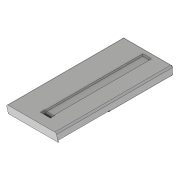
# Autodesk Inventor part: Temp
Saved by Autodesk Inventor 2021.2 (Build 252289000, 289)
## iProperties
Created: 2023-12-02
Part Number: Temp
Material: Типовые
Document SubType Name: Modeling
Designer: Egor
Density: 1 g/cm^3
Appearance: По умолчанию
Author: Egor
Autodesk Inventor part; units mm, degrees
ref_plane "YZ Plane" through (0, 0, 0) normal (1, 0, 0) x (0, 1, 0)
ref_plane "XZ Plane" through (0, 0, 0) normal (0, 1, 0) x (-1, 0, 0)
ref_plane "XY Plane" through (0, 0, 0) normal (0, 0, 1) x (1, 0, 0)
sketch "Эскиз1" plane through (0, 0, 0) normal (0, 1, 0) x (-1, 0, 0)
  line L0 (0, -50) -> (58, -50)
  line L1 (-2, -2) -> (-2, -48)
  line L2 (58, 0) -> (0, 0)
  line L3 (60, -48) -> (60, -2)
  line L4 (-2, 0) -> (60, 0)
  line L5 (60, 0) -> (60, -50)
  line L6 (60, -50) -> (-2, -50)
  line L7 (-2, -50) -> (-2, 0)
  circle A0 centre (2, -4) radius 1.6
  circle A1 centre (55, -4) radius 1.6
  circle A2 centre (55, -46) radius 1.6
  circle A3 centre (2, -46) radius 1.6
  circle A4 centre (2, -4) radius 1.6
  circle A5 centre (55, -4) radius 1.6
  circle A6 centre (55, -46) radius 1.6
  circle A7 centre (2, -46) radius 1.6
  circle A8 centre (2, -4) radius 2.4
  circle A9 centre (2, -4) radius 4
  circle A10 centre (55, -4) radius 4
  circle A11 centre (55, -4) radius 2.4
  circle A12 centre (55, -46) radius 4
  circle A13 centre (55, -46) radius 2.4
  circle A14 centre (2, -46) radius 4
  circle A15 centre (2, -46) radius 2.4
  dimension "d0" = 4.8
  dimension "d1" = 8
  dimension "d2" = 4.8
  dimension "d3" = 8
  dimension "d4" = 4.8
  dimension "d5" = 8
  dimension "d6" = 4.8
  dimension "d7" = 8
  constraints: 16 centre point, 16 end point, 9 coincident, 4 concentric, 2 parallel, 1 horizontal, 1 perpendicular, 1 point on line
  measures "d0" diameter of A8
  measures "d1" diameter of A9
  measures "d2" diameter of A11
  measures "d3" diameter of A10
  measures "d4" diameter of A13
  measures "d5" diameter of A12
  measures "d6" diameter of A15
  measures "d7" diameter of A14
extrude "Выдавливание1" add sketch "Эскиз1" along normal blind 2.5 contours L6 L7 L1 A14 L0 | A12 | A10 | A14 L1 A9 L2 L4 L5 L3 L6 L0 | A14 | L1 L7 L4 L2 A9 | A9 | A0 | A1 | A2 | A3 | A8 | A11 | A13 | A15
extrude "Выдавливание2" add sketch "Эскиз1" along normal blind 8.5 contours A12 | A10 | A14 | A9
sketch "Эскиз2" plane through (0, 0, 0) normal (0, -1, 0) x (1, 0, 0)
  line L0 (-60, 0) -> (2, 0) projected
  line L1 (2, 0) -> (2, -50) projected
  line L2 (2, -50) -> (-60, -50) projected
  line L3 (-60, -50) -> (-60, 0) projected
  line L4 (2, 0) -> (2, -50) projected
  line L5 (2.5, -50.5) -> (-60.5, -50.5)
  line L6 (-60.5, -50.5) -> (-60.5, 0.5)
  line L7 (-60.5, 0.5) -> (2.5, 0.5)
  line L8 (2.5, 0.5) -> (2.5, -50.5)
  line L9 (5, -50.5) -> (5, -53)
  line L10 (5, -53) -> (2.5, -53)
  line L11 (5, -53) -> (-63, -53)
  line L12 (-63, -53) -> (-63, 3)
  line L13 (-63, 3) -> (5, 3)
  line L14 (5, 3) -> (5, -53)
  point P0 (0, 0)
  dimension "d14" = 63
  dimension "d15" = 51
  dimension "d16" = 2.5
  dimension "d17" = 2.5
  dimension "d18" = 68
  dimension "d19" = 56
  constraints: 20 end point, 4 parallel, 2 horizontal, 2 perpendicular
  measures "d14" distance of L6.end L7.end
  measures "d15" distance of L5.end L6.end
  measures "d16" distance of L9.end L10.end
  measures "d17" distance of L9.start L9.end
  measures "d18" distance of L12.end L13.end
  measures "d19" distance of L11.end L12.end
extrude "Выдавливание3" add sketch "Эскиз2" against normal blind 2.5 contours L5 L6 L7 L8
extrude "Выдавливание4" add sketch "Эскиз2" against normal blind 35 contours L9 L10 L11 L12 L13 L14
sketch "Эскиз3" plane through (-63, 0, 3) normal (0, 0, 1) x (1, 0, 0)
  line L0 (0, 0) -> (0, 35) projected
  line L1 (0, 35) -> (68, 35)
  line L2 (68, 35) -> (68, 50)
  line L3 (68, 50) -> (0, 50)
  line L4 (0, 50) -> (0, 35)
  point P0 (63, 0)
  dimension "d24" = 15
  constraints: 8 end point, 2 parallel, 1 horizontal, 1 perpendicular
  measures "d24" distance of L2.end L1.end
extrude "Выдавливание5" add sketch "Эскиз3" against normal blind 150
sketch "Эскиз4" plane through (-63, 50, 3) normal (0, 1, 0) x (1, 0, 0)
  line L0 (0, 0) -> (0, 56) projected
  line L1 (68, 0) -> (68, 150) projected
  line L2 (0, 0) -> (68, 0)
  line L3 (68, 0) -> (68, 150)
  line L4 (68, 150) -> (0, 150)
  line L5 (0, 150) -> (0, 0)
  point P0 (63, 3)
  constraints: 8 end point, 2 parallel, 1 horizontal, 1 perpendicular
extrude "Выдавливание6" cut sketch "Эскиз4" against normal blind 2.5
sketch "Эскиз5" plane through (-63, 47.5, 3) normal (0, 1, 0) x (1, 0, 0)
  line L0 (0, 56) -> (0, 150) projected
  line L1 (0, 150) -> (10, 150)
  line L2 (10, 150) -> (10, 140)
  line L3 (10, 140) -> (0, 140)
  line L4 (0, 140) -> (0, 150)
  line L5 (68, 150) -> (0, 150) projected
  line L6 (68, 150) -> (58, 150)
  line L7 (58, 150) -> (58, 140)
  line L8 (58, 140) -> (68, 140)
  line L9 (68, 140) -> (68, 150)
  line L10 (0, 0) -> (0, 56) projected
  line L11 (0, 0) -> (10, 0)
  line L12 (10, 0) -> (10, 10)
  line L13 (10, 10) -> (0, 10)
  line L14 (0, 10) -> (0, 0)
  line L15 (10, 10) -> (58, 10)
  line L16 (58, 10) -> (58, 140)
  line L17 (58, 140) -> (10, 140)
  line L18 (10, 140) -> (10, 10)
  point P0 (63, 3)
  dimension "d29" = 10
  dimension "d30" = 10
  dimension "d31" = 10
  dimension "d32" = 10
  dimension "d33" = 10
  dimension "d34" = 10
  constraints: 32 end point, 8 parallel, 4 horizontal, 4 perpendicular
  measures "d29" distance of L2.end L3.end
  measures "d30" distance of L1.end L2.end
  measures "d31" distance of L8.end L7.end
  measures "d32" distance of L7.end L6.end
  measures "d33" distance of L13.end L12.end
  measures "d34" distance of L12.end L11.end
extrude "Выдавливание7" cut sketch "Эскиз5" against normal blind 10 contours L17 L16 L15 L18
sketch "Эскиз6" plane through (-63, 37.5, 3) normal (0, 1, 0) x (1, 0, 0)
  line L0 (58, 140) -> (10, 140) projected
  line L1 (10, 140) -> (10, 10) projected
  line L2 (10, 10) -> (58, 10) projected
  line L3 (58, 10) -> (58, 140) projected
  line L4 (0, 150) -> (68, 150) projected
  line L5 (68, 150) -> (68, 0) projected
  line L6 (68, 0) -> (0, 0) projected
  line L7 (0, 0) -> (0, 150) projected
  line L8 (68, 56) -> (0, 56) projected
  line L9 (0, 56) -> (10, 56)
  line L10 (10, 56) -> (10, 46)
  line L11 (10, 46) -> (0, 46)
  line L12 (0, 46) -> (0, 56)
  line L13 (10, 46) -> (58, 46)
  line L14 (58, 46) -> (58, 10)
  line L15 (58, 10) -> (10, 10)
  line L16 (10, 10) -> (10, 46)
  point P0 (63, 3)
  dimension "d37" = 10
  dimension "d38" = 10
  constraints: 16 end point, 4 parallel, 2 horizontal, 2 perpendicular
  measures "d37" distance of L10.end L11.end
  measures "d38" distance of L9.end L10.end
extrude "Выдавливание8" cut sketch "Эскиз6" against normal blind 10 contours L3 L2 L1 L13
sketch "Эскиз7" plane through (-63, 47.5, 3) normal (0, 1, 0) x (1, 0, 0)
  line L0 (0, 0) -> (0, 150) projected
  line L1 (0, 150) -> (2.5, 150)
  line L2 (2.5, 150) -> (2.5, 147.5)
  line L3 (2.5, 147.5) -> (0, 147.5)
  line L4 (0, 147.5) -> (0, 150)
  line L5 (68, 150) -> (68, 0) projected
  line L6 (68, 150) -> (65.5, 150)
  line L7 (65.5, 150) -> (65.5, 147.5)
  line L8 (65.5, 147.5) -> (68, 147.5)
  line L9 (68, 147.5) -> (68, 150)
  line L10 (2.5, 2.5) -> (2.5, 53.5) projected
  line L11 (65.5, 147.5) -> (2.5, 147.5)
  line L12 (2.5, 147.5) -> (2.5, 10)
  line L13 (2.5, 10) -> (65.5, 10)
  line L14 (65.5, 10) -> (65.5, 147.5)
  point P0 (63, 3)
  dimension "d41" = 2.5
  dimension "d42" = 2.5
  dimension "d43" = 2.5
  dimension "d44" = 2.5
  dimension "d45" = 137.5
  constraints: 24 end point, 6 parallel, 3 horizontal, 3 perpendicular, 1 point on line
  measures "d41" distance of L2.end L3.end
  measures "d42" distance of L1.end L2.end
  measures "d43" distance of L8.end L7.end
  measures "d44" distance of L7.end L6.end
  measures "d45" distance of L12.end L11.end
extrude "Выдавливание9" cut sketch "Эскиз7" against normal blind 10 contours L11 L14 L13 L10 L12
sketch "Эскиз8" plane through (-63, 37.5, 3) normal (0, 1, 0) x (1, 0, 0)
  line L0 (58, 10) -> (58, 46) projected
  line L1 (58, 46) -> (10, 46) projected
  line L2 (10, 46) -> (10, 10) projected
  line L3 (2.5, 10) -> (10, 10) projected
  line L4 (2.5, 147.5) -> (2.5, 10) projected
  line L5 (65.5, 147.5) -> (2.5, 147.5) projected
  line L6 (65.5, 10) -> (65.5, 147.5) projected
  line L7 (58, 10) -> (65.5, 10) projected
  line L8 (10, 10) -> (58, 10) projected
  line L9 (0, 150) -> (68, 150) projected
  line L10 (68, 150) -> (68, 0) projected
  line L11 (68, 0) -> (0, 0) projected
  line L12 (0, 0) -> (0, 150) projected
  circle A0 centre (8, 49) radius 2.4 projected
  line L13 (2.5, 53.5) -> (65.5, 53.5) projected
  line L14 (65.5, 147.5) -> (65.5, 10) projected
  circle A1 centre (61, 49) radius 4 projected
  circle A2 centre (8, 7) radius 4 projected
  circle A3 centre (8, 49) radius 4 projected
  line L15 (2.5, 2.5) -> (65.5, 2.5) projected
  line L16 (65.5, 2.5) -> (65.5, 53.5) projected
  line L17 (65.5, 53.5) -> (2.5, 53.5) projected
  line L18 (2.5, 53.5) -> (2.5, 2.5) projected
  circle A4 centre (61, 7) radius 4 projected
  circle A5 centre (8, 7) radius 4 projected
  line L19 (2.5, 2.5) -> (2.5, 53.5) projected
  line L20 (65.5, 2.5) -> (2.5, 2.5) projected
  line L21 (65.5, 53.5) -> (65.5, 2.5) projected
  circle A6 centre (61, 7) radius 2.4 projected
  line L22 (2.5, 53.5) -> (65.5, 53.5)
  line L23 (65.5, 53.5) -> (65.5, 2.5)
  line L24 (65.5, 2.5) -> (2.5, 2.5)
  line L25 (2.5, 2.5) -> (2.5, 53.5)
  point P0 (63, 3)
  point P1 (58.3542, 10)
  point P2 (63.6458, 10)
  point P3 (10.6458, 10)
  point P4 (10, 10.4641)
  point P5 (10, 45.5359)
  point P6 (10.6458, 46)
  constraints: 8 end point, 2 parallel, 1 horizontal, 1 perpendicular
extrude "Выдавливание10" cut sketch "Эскиз8" along normal mid plane 20 contours L0 L1 A3 L2 A2 L3 L4 L13 L6 L7 A4 | L7 A4 L16 L15 L18 L3 A2 L8 | A4 L7 | L7 A4 | A2 L3 L8 | L8 L2 A2 | A3 L2 L1 | L1 L2 A3 | L3 A2 L2 | A0 | A1 | A6
sketch "Эскиз9" plane through (-63, 0, 3) normal (0, 0, 1) x (1, 0, 0)
  line L0 (68, 0) -> (68, 47.5) projected
  line L1 (68, 35) -> (0, 35) projected
  line L2 (68, 47.5) -> (0, 47.5)
  line L3 (0, 47.5) -> (0, 35)
  line L4 (0, 35) -> (68, 35)
  line L5 (68, 35) -> (68, 47.5)
  point P0 (63, 0)
  constraints: 8 end point, 2 parallel, 1 horizontal, 1 perpendicular
extrude "Выдавливание11" add sketch "Эскиз9" along normal blind 10
sketch "Эскиз12" plane through (-63, 37.5, 3) normal (0, 1, 0) x (1, 0, 0)
  line L0 (65.5, 2.5) -> (65.5, 53.5) projected
  line L1 (65.5, 53.5) -> (55.5, 53.5)
  line L2 (55.5, 53.5) -> (55.5, 63.5)
  line L3 (55.5, 63.5) -> (65.5, 63.5)
  line L4 (65.5, 63.5) -> (65.5, 53.5)
  line L5 (2.5, 53.5) -> (2.5, 2.5) projected
  line L6 (2.5, 53.5) -> (12.5, 53.5)
  line L7 (12.5, 53.5) -> (12.5, 63.5)
  line L8 (12.5, 63.5) -> (2.5, 63.5)
  line L9 (2.5, 63.5) -> (2.5, 53.5)
  point P0 (63, 3)
  dimension "d52" = 10
  dimension "d53" = 10
  dimension "d54" = 10
  constraints: 16 end point, 4 parallel, 2 horizontal, 2 perpendicular
  measures "d52" distance of L2.end L3.end
  measures "d53" distance of L1.end L2.end
  measures "d54" distance of L8.end L7.end
extrude "Выдавливание12" add sketch "Эскиз12" along normal blind 10
sketch "Эскиз16" plane through (0, 0, 0) normal (0, -1, 0) x (1, 0, 0)
  line L0 (5, -53) -> (5, 3) projected
  line L1 (-63, -53) -> (5, -53) projected
  line L2 (5, 3) -> (-63, 3)
  line L3 (-63, 3) -> (-63, -53)
  line L4 (-63, -53) -> (5, -53)
  line L5 (5, -53) -> (5, 3)
  line L6 (-63, -147) -> (-63, 13) projected
  line L7 (5, -53) -> (-63, -53)
  line L8 (-63, -53) -> (-63, -60)
  line L9 (-63, -60) -> (5, -60)
  line L10 (5, -60) -> (5, -53)
  line L11 (-63, 3) -> (-63, -53) projected
  line L12 (5, -147) -> (5, 13) projected
  line L13 (-63, 3) -> (5, 3)
  line L14 (5, 3) -> (5, 10)
  line L15 (5, 10) -> (-63, 10)
  line L16 (-63, 10) -> (-63, 3)
  point P0 (0, 0)
  dimension "d59" = 7
  dimension "d60" = 7
  constraints: 24 end point, 6 parallel, 3 horizontal, 3 perpendicular, 2 point on line
  measures "d59" distance of L8.end L7.end
  measures "d60" distance of L14.end L13.end
extrude "Выдавливание13" cut sketch "Эскиз16" against normal blind 37.5
sketch "Эскиз17" plane through (-63, 47.5, 3) normal (0, 1, 0) x (1, 0, 0)
  line L0 (68, -10) -> (0, -10)
  line L1 (0, -10) -> (0, 150)
  line L2 (0, 150) -> (68, 150)
  line L3 (68, 150) -> (68, -10)
  line L4 (45.5, 63.5) -> (45.5, 127.5)
  line L5 (2.5, 147.5) -> (65.5, 147.5) projected
  line L6 (45.5, 127.5) -> (45.5, 132.5)
  line L7 (33.5, 132.5) -> (33.5, 7.5)
  line L8 (33.5, 7.5) -> (45.5, 7.5)
  line L9 (45.5, 7.5) -> (45.5, 63.5)
  line L10 (33.5, 132.5) -> (32, 132.5)
  line L11 (32, 132.5) -> (32, 134)
  line L12 (32, 134) -> (33.5, 134)
  line L13 (33.5, 134) -> (33.5, 132.5)
  line L14 (45.5, 7.5) -> (47, 7.5)
  line L15 (47, 7.5) -> (47, 6)
  line L16 (47, 6) -> (45.5, 6)
  line L17 (45.5, 6) -> (45.5, 7.5)
  line L18 (47, 6) -> (32, 6)
  line L19 (32, 6) -> (32, 134)
  line L20 (47, 134) -> (47, 6)
  line L21 (45.5, 134) -> (45.5, 132.5)
  line L22 (33.5, 132.5) -> (33.5, 134)
  line L23 (47, 134) -> (47, 144)
  line L24 (47, 144) -> (32, 144)
  line L25 (32, 144) -> (32, 134)
  line L26 (33.5, 134) -> (32, 134)
  line L27 (32, 134) -> (32, 144)
  line L28 (32, 144) -> (33.5, 144)
  line L29 (33.5, 144) -> (33.5, 134)
  line L30 (45.5, 134) -> (47, 134)
  line L31 (47, 134) -> (47, 144)
  line L32 (47, 144) -> (45.5, 144)
  line L33 (45.5, 144) -> (45.5, 134)
  line L34 (32, 144) -> (47, 144)
  line L35 (47, 144) -> (47, 142.5)
  line L36 (47, 142.5) -> (32, 142.5)
  line L37 (32, 142.5) -> (32, 144)
  line L38 (32, 6) -> (47, 6)
  line L39 (47, 6) -> (47, 7.5)
  line L40 (47, 7.5) -> (32, 7.5)
  line L41 (32, 7.5) -> (32, 6)
  point P0 (63, 3)
  point P1 (55.5, 63.5)
  point P2 (33.5, 142.5)
  point P3 (45.5, 142.5)
  dimension "d64" = 64
  dimension "d65" = 5
  dimension "d66" = 12
  dimension "d67" = 125
  dimension "d68" = 1.5
  dimension "d69" = 1.5
  dimension "d70" = 1.5
  dimension "d71" = 1.5
  dimension "d72" = 10
  dimension "d73" = 1.5
  constraints: 82 end point, 17 parallel, 11 perpendicular, 8 horizontal, 3 point on line
  measures "d64" distance of L4.start L4.end
  measures "d65" distance of L4.end L6.end
  measures "d66" distance of L6.end L7.start
  measures "d67" distance of L7.start L7.end
  measures "d68" distance of L11.end L12.end
  measures "d69" distance of L10.end L11.end
  measures "d70" distance of L15.end L16.end
  measures "d71" distance of L14.end L15.end
  measures "d72" distance of L23.end L23.start
  measures "d73" distance of L34.end L35.end
extrude "Выдавливание14" add sketch "Эскиз17" against normal up to surface (10 mm away) contours L4 L6 L21 L30 L20 L14 L9 | L40 L19 L10 L7 | L33 L36 L23 L30 | L10 L11 L12 L13 | L36 L29 L24 L33 | L33 L24 L23 L36 | L12 L25 L36 L29 | L36 L25 L24 L29
sketch "Эскиз18" plane through (-63, 37.5, 3) normal (0, 1, 0) x (1, 0, 0)
  line L0 (45.5, 142.5) -> (45.5, 7.5) projected
  line L1 (33.5, 142.5) -> (45.5, 142.5)
  line L2 (45.5, 142.5) -> (45.5, 7.5)
  line L3 (45.5, 7.5) -> (33.5, 7.5)
  line L4 (33.5, 7.5) -> (33.5, 142.5)
  point P0 (63, 3)
  constraints: 8 end point, 2 parallel, 1 horizontal, 1 perpendicular
extrude "Выдавливание15" add sketch "Эскиз18" along normal blind 7.5
sketch "Эскиз19" plane through (-63, 47.5, 3) normal (0, 1, 0) x (1, 0, 0)
  line L0 (68, 150) -> (0, 150) projected
  line L1 (68, 150) -> (68, -10) projected
  line L2 (0, 150) -> (68, 150)
  line L3 (68, 150) -> (68, -10)
  line L4 (68, -10) -> (0, -10)
  line L5 (0, -10) -> (0, 150)
  point P0 (63, 3)
  constraints: 8 end point, 2 parallel, 1 horizontal, 1 perpendicular
sketch "Эскиз20" plane through (-63, 37.5, 3) normal (0, 1, 0) x (1, 0, 0)
  line L0 (2.5, 147.5) -> (65.5, 147.5) projected
  line L1 (32, 63) -> (32, 7.5) projected
  line L2 (2.5, 147.5) -> (32, 147.5)
  line L3 (32, 147.5) -> (32, 63)
  line L4 (32, 63) -> (2.5, 63)
  line L5 (2.5, 63) -> (2.5, 147.5)
  line L6 (47, 7.5) -> (47, 144) projected
  line L7 (32, 147.5) -> (47, 147.5)
  line L8 (47, 147.5) -> (47, 144)
  line L9 (47, 144) -> (32, 144)
  line L10 (32, 144) -> (32, 147.5)
  line L11 (47, 147.5) -> (65.5, 147.5)
  line L12 (65.5, 147.5) -> (65.5, 63)
  line L13 (65.5, 63) -> (47, 63)
  line L14 (47, 63) -> (47, 147.5)
  point P0 (63, 3)
  constraints: 24 end point, 6 parallel, 3 horizontal, 3 perpendicular, 1 point on line
extrude "Выдавливание16" add sketch "Эскиз20" along normal blind 10
sketch "Эскиз21" plane through (-63, 47.5, 3) normal (0, 1, 0) x (1, 0, 0)
  line L0 (12.5, 63) -> (32, 63) projected
  line L1 (65.5, 2.5) -> (2.5, 2.5) projected
  line L2 (32, 63) -> (2.5, 63)
  line L3 (2.5, 63) -> (2.5, 2.5)
  line L4 (2.5, 2.5) -> (32, 2.5)
  line L5 (32, 2.5) -> (32, 63)
  line L6 (47, 63) -> (55.5, 63) projected
  line L7 (65.5, 53.5) -> (65.5, 2.5) projected
  line L8 (47, 63) -> (65.5, 63)
  line L9 (65.5, 63) -> (65.5, 2.5)
  line L10 (65.5, 2.5) -> (47, 2.5)
  line L11 (47, 2.5) -> (47, 63)
  line L12 (32, 2.5) -> (47, 2.5)
  line L13 (47, 2.5) -> (47, 5.5)
  line L14 (47, 5.5) -> (32, 5.5)
  line L15 (32, 5.5) -> (32, 2.5)
  point P0 (63, 3)
  dimension "d80" = 3
  constraints: 24 end point, 6 parallel, 3 horizontal, 3 perpendicular, 1 point on line
  measures "d80" distance of L13.end L12.end
extrude "Выдавливание17" add sketch "Эскиз21" against normal blind 10
sketch "Эскиз22" plane through (0, 37.5, 0) normal (0, -1, 0) x (1, 0, 0)
  line L0 (-16, -4.5) -> (-16, -2.5) projected
  line L1 (-16, -2.5) -> (-31, -2.5)
  line L2 (-31, -2.5) -> (-31, 0)
  line L3 (-31, 0) -> (-16, 0)
  line L4 (-16, 0) -> (-16, -2.5)
  point P0 (0, 0)
  constraints: 8 end point, 2 parallel, 1 horizontal, 1 perpendicular
extrude "Выдавливание18" cut sketch "Эскиз22" against normal blind 10
sketch "Эскиз23" plane through (-63, 47.5, 3) normal (0, 1, 0) x (1, 0, 0)
  line L0 (33.5, 7.5) -> (45.5, 7.5) projected
  line L1 (45.5, 142.5) -> (45.5, 7.5) projected
  line L2 (33.5, 7.5) -> (45.5, 7.5)
  line L3 (45.5, 7.5) -> (45.5, 9.5)
  line L4 (45.5, 9.5) -> (33.5, 9.5)
  line L5 (33.5, 9.5) -> (33.5, 7.5)
  point P0 (63, 3)
  dimension "d85" = 2
  constraints: 8 end point, 2 parallel, 1 horizontal, 1 perpendicular, 1 point on line
  measures "d85" distance of L3.end L2.end
extrude "Выдавливание19" cut sketch "Эскиз23" against normal blind 10
sketch "Эскиз24" plane through (-63, 47.5, 3) normal (0, 1, 0) x (1, 0, 0)
  line L0 (32, 7.5) -> (33.5, 7.5) projected
  line L1 (47, 3) -> (32, 3) projected
  line L2 (33.5, 7.5) -> (32, 7.5)
  line L3 (32, 7.5) -> (32, 3)
  line L4 (32, 3) -> (33.5, 3)
  line L5 (33.5, 3) -> (33.5, 7.5)
  line L6 (45.5, 7.5) -> (47, 7.5) projected
  line L7 (45.5, 7.5) -> (47, 7.5)
  line L8 (47, 7.5) -> (47, 3)
  line L9 (47, 3) -> (45.5, 3)
  line L10 (45.5, 3) -> (45.5, 7.5)
  point P0 (63, 3)
  constraints: 16 end point, 4 parallel, 2 horizontal, 2 perpendicular, 1 point on line
extrude "Выдавливание20" add sketch "Эскиз24" against normal blind 10
sketch "Эскиз25" plane through (-63, 47.5, 3) normal (0, 1, 0) x (1, 0, 0)
  line L0 (33.5, 3) -> (33.5, 142.5) projected
  line L1 (45.5, 142.5) -> (45.5, 3) projected
  line L2 (33.5, 3) -> (45.5, 3)
  line L3 (45.5, 3) -> (45.5, 10.5)
  line L4 (45.5, 10.5) -> (33.5, 10.5)
  line L5 (33.5, 10.5) -> (33.5, 3)
  point P0 (63, 3)
  dimension "d90" = 7.5
  constraints: 8 end point, 2 parallel, 1 horizontal, 1 perpendicular, 1 point on line
  measures "d90" distance of L3.end L2.end
extrude "Выдавливание21" add sketch "Эскиз25" against normal blind 1
sketch "Эскиз26" plane through (0, 37.5, 0) normal (0, -1, 0) x (1, 0, 0)
  point P0 (0, 0)
sketch "Эскиз27" plane through (0, 37.5, 0) normal (0, -1, 0) x (1, 0, 0)
  line L0 (-29.5, 0) -> (-29.5, -6.5) projected
  line L1 (-29.5, -6.5) -> (-17.5, -6.5) projected
  line L2 (-17.5, -6.5) -> (-17.5, 0) projected
  line L3 (-17.5, 0) -> (-29.5, 0) projected
  line L4 (-63, -60) -> (5, -60) projected
  line L5 (5, 10) -> (5, -60) projected
  line L6 (5, 13) -> (5, 10) projected
  line L7 (-63, 13) -> (5, 13) projected
  line L8 (-63, 10) -> (-63, 13) projected
  line L9 (5, 10) -> (-63, 10) projected
  line L10 (-63, -60) -> (-63, 10) projected
  line L11 (-63, -147) -> (-63, -60) projected
  line L12 (5, -147) -> (-63, -147) projected
  line L13 (5, -60) -> (5, -147) projected
  line L14 (5, 10) -> (-2, 10)
  line L15 (-2, 10) -> (-2, 3)
  line L16 (-2, 3) -> (5, 3)
  line L17 (5, 3) -> (5, 10)
  line L18 (-63, 10) -> (-56, 10)
  line L19 (-56, 10) -> (-56, 3)
  line L20 (-56, 3) -> (-63, 3)
  line L21 (-63, 3) -> (-63, 10)
  line L22 (-63, -60) -> (-56, -60)
  line L23 (-56, -60) -> (-56, -53)
  line L24 (-56, -53) -> (-63, -53)
  line L25 (-63, -53) -> (-63, -60)
  line L26 (5, -60) -> (-63, -60) projected
  line L27 (5, -60) -> (-2, -60)
  line L28 (-2, -60) -> (-2, -53)
  line L29 (-2, -53) -> (5, -53)
  line L30 (5, -53) -> (5, -60)
  circle A0 centre (-2, -56.5) radius 2.4
  circle A1 centre (-56, -56.5) radius 2.4
  circle A2 centre (-56, 6.5) radius 2.4
  circle A3 centre (-2, 6.5) radius 2.4
  point P0 (0, 0)
  dimension "d93" = 7
  dimension "d94" = 7
  dimension "d95" = 7
  dimension "d96" = 7
  dimension "d97" = 4.8
  constraints: 32 end point, 8 parallel, 4 centre point, 4 horizontal, 4 midpoint, 4 perpendicular, 4 point on line
  measures "d93" distance of L16.end L15.end
  measures "d94" distance of L15.end L14.end
  measures "d95" distance of L19.end L20.end
  measures "d96" distance of L23.end L22.end
  measures "d97" diameter of A0
extrude "Выдавливание22" cut sketch "Эскиз27" against normal blind 6 contours A1 L23 | L23 A1 | A0 L28 | L28 A0 | A2 L19 | L19 A2 | A3 L15 | L15 A3
sketch "Эскиз28" plane through (5, 35, -147) normal (1, 0, 0) x (0, 0, -1)
  line L0 (-160, 0) -> (-160, 12.5)
  line L1 (-150, -35) -> (-160, 0)
  line L2 (-150, -35) -> (-160, 12.5)
  line L3 (-160, 0) -> (-150, -35)
  line L4 (-160, 12.5) -> (-160, 0) projected
  line L5 (0, 12.5) -> (-160, 12.5) projected
  point P0 (-147, -35)
  constraints: 8 end point
extrude "Выдавливание23" cut sketch "Эскиз28" against normal through all
fillet "Сопряжение1" radius 2 8 edges at (5, 47.5, -67) (-29, 47.5, -147) (-63, 47.5, -67) (5, 41.25, -147) (-63, 41.25, -147) (-29, 35, -147) (5, 35, -103.5) (-63, 35, -103.5)
fillet "Сопряжение2" radius 2 1 edges at (-23.5, 45, -6.5)
fillet "Сопряжение3" radius 2 4 edges at (-23.5, 37.5, -6.5) (-17.5, 37.5, -3.25) (-29.5, 37.5, -3.25) (-23.5, 37.5, 0)
sketch "Эскиз29" plane through (0, 37.5, 0) normal (0, -1, 0) x (1, 0, 0)
  line L0 (-31.5, -8.5) -> (-29.5, -6.5) projected
  line L1 (-31.5, -8.5) -> (-31.5, -28.5)
  line L2 (-31.5, -28.5) -> (-15.5, -28.5)
  line L3 (-15.5, -28.5) -> (-15.5, -22.5)
  line L4 (-15.5, -22.5) -> (-31.5, -22.5)
  line L5 (-31.5, -28.5) -> (-28.5, -28.5)
  line L6 (-28.5, -28.5) -> (-28.5, -22.5)
  line L7 (-28.5, -22.5) -> (-31.5, -22.5)
  line L8 (-31.5, -22.5) -> (-31.5, -28.5)
  point P0 (0, 0)
  dimension "d105" = 20
  dimension "d106" = 3
  constraints: 16 end point, 3 perpendicular, 2 horizontal, 2 parallel, 2 point on line, 1 vertical
  measures "d105" distance of L0.start L1.end
  measures "d106" distance of L7.end L6.end
extrude "Выдавливание24" add sketch "Эскиз29" along normal blind 5 contours L4 L6 L2 L1
sketch "Эскиз30" plane through (0, 32.5, 0) normal (0, -1, 0) x (1, 0, 0)
  line L0 (-31.5, -28.5) -> (-31.5, -22.5) projected
  line L1 (-31.5, -28.5) -> (-16.5, -28.5)
  line L2 (-16.5, -28.5) -> (-16.5, -22.5)
  line L3 (-16.5, -22.5) -> (-31.5, -22.5)
  line L4 (-31.5, -22.5) -> (-31.5, -28.5)
  point P0 (0, 0)
  dimension "d109" = 15
  constraints: 8 end point, 2 parallel, 1 horizontal, 1 perpendicular
  measures "d109" distance of L3.end L2.end
extrude "Выдавливание25" add sketch "Эскиз30" against normal blind 2
fillet "Сопряжение4" radius 1 13 edges at (-28.5, 37.5, -25.5) (-30, 37.5, -22.5) (-31.5, 37.5, -25.5) (-30, 37.5, -28.5) (-31.5, 32.5, -25.5) (-24, 32.5, -22.5) (-24, 32.5, -28.5) (-16.5, 32.5, -25.5) (-28.5, 34.5, -25.5) (-31.5, 35, -22.5) (-28.5, 36, -22.5) (-28.5, 36, -28.5) (-31.5, 35, -28.5)
sketch "Эскиз31" plane through (-63, 47.5, 3) normal (0, 1, 0) x (1, 0, 0)
  line L0 (45.5, 3) -> (45.5, 10.5) projected
  line L1 (33.5, 9.5) -> (33.5, 3) projected
  line L2 (45.5, 10.5) -> (33.5, 10.5)
  line L3 (33.5, 10.5) -> (33.5, 5.5)
  line L4 (33.5, 5.5) -> (45.5, 5.5)
  line L5 (45.5, 5.5) -> (45.5, 10.5)
  point P0 (63, 3)
  point P1 (45.5, 5.5)
  dimension "d113" = 5
  constraints: 8 end point, 2 parallel, 1 horizontal, 1 perpendicular, 1 point on line
  measures "d113" distance of L3.end L2.end
extrude "Выдавливание26" cut sketch "Эскиз31" against normal blind 2
sketch "Эскиз32" plane through (-63, 47.5, 3) normal (0, 1, 0) x (1, 0, 0)
  line L0 (33.5, 5.5) -> (45.5, 5.5) projected
  line L1 (32.5, 3.5) -> (46.5, 3.5)
  line L2 (46.5, 3.5) -> (46.5, 9.5)
  line L3 (46.5, 9.5) -> (32.5, 9.5)
  line L4 (32.5, 9.5) -> (32.5, 3.5)
  point P0 (63, 3)
  dimension "d118" = 14
  constraints: 8 end point, 2 parallel, 1 horizontal, 1 perpendicular
  measures "d118" distance of L3.end L2.end
extrude "Выдавливание27" cut sketch "Эскиз32" against normal blind 1
sketch "Эскиз33" plane through (0, 32.5, 0) normal (0, -1, 0) x (1, 0, 0)
  line L0 (-35.6143, -40.4907) -> (-11.0678, -40.4907)
  line L1 (-11.0678, -40.4907) -> (-11.0678, -15.5059)
  line L2 (-11.0678, -15.5059) -> (-35.6143, -15.5059)
  line L3 (-35.6143, -15.5059) -> (-35.6143, -40.4907)
  point P0 (0, 0)
  constraints: 8 end point, 2 parallel, 1 horizontal, 1 perpendicular
extrude "Выдавливание28" cut sketch "Эскиз33" against normal up to surface (5 mm away)
